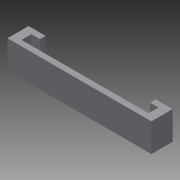
# Autodesk Inventor part: Side Grapper
Saved by Autodesk Inventor 2015 (Build 190159000, 159)
## iProperties
Created: 2016-05-27
Part Number: Side Grapper
Material: Generic
Document SubType Name: Modeling
Designer: Toby
Density: 1 g/cm^3
Appearance: Default
Author: Toby
Autodesk Inventor part; units mm, degrees
ref_plane "YZ Plane" through (0, 0, 0) normal (1, 0, 0) x (0, 1, 0)
ref_plane "XZ Plane" through (0, 0, 0) normal (0, 1, 0) x (-1, 0, 0)
ref_plane "XY Plane" through (0, 0, 0) normal (0, 0, 1) x (1, 0, 0)
sketch "Sketch1" plane through (0, 0, 0) normal (0, 0, 1) x (1, 0, 0)
  line L0 (-25.6928, -3.3339) -> (25.3072, -3.3339)
  line L1 (25.3072, -3.3339) -> (25.3072, -5.3339)
  line L2 (25.3072, -5.3339) -> (-25.6928, -5.3339)
  line L3 (-25.6928, -5.3339) -> (-25.6928, -3.3339)
  line L4 (-25.6928, -5.3339) -> (-22.6928, -5.3339)
  line L5 (-22.6928, -5.3339) -> (-22.6928, 2.1661)
  line L6 (-22.6928, 2.1661) -> (-25.6928, 2.1661)
  line L7 (-25.6928, 2.1661) -> (-25.6928, -5.3339)
  line L8 (-25.6928, 2.1661) -> (-19.6928, 2.1661)
  line L9 (-19.6928, 2.1661) -> (-19.6928, 0.1661)
  line L10 (-19.6928, 0.1661) -> (-25.6928, 0.1661)
  line L11 (-25.6928, 0.1661) -> (-25.6928, 2.1661)
  line L12 (25.3072, -5.3339) -> (22.3072, -5.3339)
  line L13 (22.3072, -5.3339) -> (22.3072, 2.1661)
  line L14 (22.3072, 2.1661) -> (25.3072, 2.1661)
  line L15 (25.3072, 2.1661) -> (25.3072, -5.3339)
  line L16 (25.3072, 2.1661) -> (19.3072, 2.1661)
  line L17 (19.3072, 2.1661) -> (19.3072, 0.1661)
  line L18 (19.3072, 0.1661) -> (25.3072, 0.1661)
  line L19 (25.3072, 0.1661) -> (25.3072, 2.1661)
  point P0 (0, 0)
  dimension "d0" = 45
  dimension "d1" = 3.5
  dimension "d2" = 6
  dimension "d3" = 6
  dimension "d4" = 51
  dimension "d5" = 3
  dimension "d6" = 2
  dimension "d7" = 3
  dimension "d8" = 2
  dimension "d9" = 2
  constraints: 40 end point, 10 parallel, 5 horizontal, 5 perpendicular, 1 point on line
  measures "d0" distance between parallel lines of L13 L5
  measures "d1" distance between parallel lines of L0 L10
  measures "d2" distance of L6.end L8.end
  measures "d3" distance of L14.end L16.end
  measures "d4" distance of L0.start L0.end
  measures "d5" distance between parallel lines of L13 L15
  measures "d6" distance between parallel lines of L18 L16
  measures "d7" distance between parallel lines of L7 L5
  measures "d8" distance between parallel lines of L10 L8
  measures "d9" distance between parallel lines of L2 L0
extrude "Extrusion1" add sketch "Sketch1" along normal blind 10
body "Solid1"
